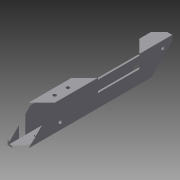
# Autodesk Inventor part: Fender Side Right
Saved by Autodesk Inventor 2015 (Build 190159000, 159)
## iProperties
Created: 2015-02-14
Part Number: Fender Side Right
Material: Generic
Document SubType Name: Modeling
Designer: chapale16
Density: 1 g/cm^3
Appearance: Default
Author: chapale16
Autodesk Inventor part; units mm, degrees
ref_plane "YZ Plane" through (0, 0, 0) normal (1, 0, 0) x (0, 1, 0)
ref_plane "XZ Plane" through (0, 0, 0) normal (0, 1, 0) x (-1, 0, 0)
ref_plane "XY Plane" through (0, 0, 0) normal (0, 0, 1) x (1, 0, 0)
sketch "Sketch1" plane through (0, 0, 0) normal (0, 0, 1) x (1, 0, 0)
  line L0 (0, 0) -> (25.4, 0)
  line L1 (25.4, 0) -> (25.4, 50.8)
  line L2 (25.4, 50.8) -> (0, 50.8)
  line L3 (0, 50.8) -> (0, 0)
  line L4 (3.175, 47.625) -> (22.225, 47.625)
  line L5 (22.225, 47.625) -> (22.225, 3.175)
  line L6 (22.225, 3.175) -> (3.175, 3.175)
  line L7 (3.175, 3.175) -> (3.175, 47.625)
  dimension "d0" = 25.4
  dimension "d1" = 50.8
  dimension "d2" = 3.175
  constraints: 16 end point, 4 parallel, 2 perpendicular, 1 horizontal, 3 other
  measures "d0" distance of L2.end L1.end
  measures "d1" distance of L1.end L0.end
  measures "d2" distance between parallel lines of L2 L4
extrude "Extrusion1" add sketch "Sketch1" along normal blind 292.1
sketch "Sketch2" plane through (0, 50.8, 0) normal (0, 1, 0) x (1, 0, 0)
  line L0 (25.4, 0) -> (25.4, -292.1) projected
  line L1 (0, 0) -> (0, -292.1) projected
  line L2 (25.4, -63.4492) -> (0, -38.0492)
  line L3 (25.4, -143.5862) -> (0, -168.9862)
  line L4 (0, -168.9862) -> (0, -38.0492)
  line L5 (25.4, -143.5862) -> (25.4, -63.4492)
  constraints: 8 end point, 4 point on line, 2 collinear
extrude "Extrusion2" cut sketch "Sketch2" against normal blind 25.4
sketch "Sketch3" plane through (25.4, 0, 0) normal (1, 0, 0) x (0, 0, -1)
  line L0 (-15.2442, 1674.64) -> (-15.2442, -147.81) projected
  line L1 (17.7758, 1674.64) -> (17.7758, -147.81) projected
  circle A0 centre (-215.7344, 12.9914) radius 3.175 projected
  circle A1 centre (-14.559, 38.1) radius 3.175 projected
  circle A2 centre (-14.559, 12.7) radius 3.175 projected
  line L2 (-34.8742, 50.8) -> (-34.8742, 25.4) projected
  line L3 (-34.8742, 25.4) -> (-169.9072, 25.4) projected
  line L4 (-169.9072, 25.4) -> (-169.9072, 50.8) projected
  line L5 (-169.9072, 50.8) -> (-234.7144, 50.8) projected
  line L6 (-234.7144, 50.8) -> (-234.7144, 0) projected
  line L7 (0, 0) -> (-234.7144, 0) projected
  line L8 (0, 50.8) -> (0, 0) projected
  line L9 (0, 50.8) -> (-34.8742, 50.8) projected
  line L10 (0, 0) -> (-292.1, 0) projected
  line L11 (-34.8742, 50.8) -> (17.7758, 50.8)
  line L12 (17.7758, 50.8) -> (17.7758, 0)
  line L13 (17.7758, 0) -> (-34.8742, 0)
  line L14 (-34.8742, 0) -> (-34.8742, 50.8)
  circle A3 centre (-18.3666, 38.1) radius 3.175
  circle A4 centre (-18.3666, 12.7) radius 3.175
  dimension "d7" = 6.35
  dimension "d8" = 6.35
  constraints: 8 end point, 2 centre point, 2 coincident, 2 parallel, 2 point on line, 1 horizontal, 1 perpendicular
  measures "d7" diameter of A3
  measures "d8" diameter of A4
extrude "Extrusion3" cut sketch "Sketch3" against normal blind 25.4 contours A3 L0 | L0 A3 A1 | A1 A3 | A4 L0 | L0 A4 A2 | A2 A4 picked at (-16.0741, 38.1) picked at (-16.0741, 12.7)
sketch "Sketch4" plane through (0, 50.8, 292.1) normal (0, 1, 0) x (1, 0, 0)
  circle A0 centre (12.7528, 77.8097) radius 3.175 projected
  circle A1 centre (-65.5643, -12.7) radius 3.175 projected
  circle A2 centre (16.4357, -12.7) radius 3.175 projected
  circle A3 centre (-65.5643, 77.8097) radius 3.175 projected
  line L0 (-75.3643, -25.3975) -> (26.2357, -25.3975) projected
  line L1 (26.2357, 88.0643) -> (26.2357, -25.3975) projected
  line L2 (26.2357, 88.0643) -> (-75.3643, 88.0643) projected
  line L3 (-75.3643, 88.0643) -> (-75.3643, -25.3975) projected
  circle A4 centre (-24.5643, 24.5643) radius 41 projected
  circle A5 centre (-24.6714, 70.0642) radius 2.55 projected
  circle A6 centre (-70.0642, 24.4572) radius 2.55 projected
  circle A7 centre (-24.4572, -20.9355) radius 2.55 projected
  circle A8 centre (20.9355, 24.6714) radius 2.55 projected
  circle A9 centre (7.5332, 56.8133) radius 2.55 projected
  circle A10 centre (7.6847, -7.5332) radius 2.55 projected
  circle A11 centre (-56.6619, -7.6847) radius 2.55 projected
  circle A12 centre (-56.8133, 56.6619) radius 2.55 projected
  circle A13 centre (-65.5643, 77.8097) radius 3.175 projected
  circle A14 centre (-65.5643, -12.7) radius 3.175 projected
  circle A15 centre (16.4357, -12.7) radius 3.175 projected
  circle A16 centre (-24.5643, 24.5643) radius 9.525 projected
  circle A17 centre (12.9268, 103.2097) radius 3.175 projected
  circle A18 centre (-78.1301, -12.7) radius 3.175 projected
  circle A19 centre (12.7528, 77.8097) radius 3.175 projected
  line L4 (25.4, -25.4) -> (-88.9, -25.4) projected
  line L5 (25.4, 123.9554) -> (25.4, -25.4) projected
  line L6 (25.4, 123.9554) -> (-88.9, 92.2721) projected
  line L7 (-88.9, -25.4) -> (-88.9, 92.2721) projected
  point P0 (0, 292.1)
extrude "Extrusion4" cut sketch "Sketch4" against normal blind 25.4 contours A0 | A17
sketch "Sketch5" plane through (25.4, 0, 0) normal (1, 0, 0) x (0, 0, -1)
  line L0 (-292.1, 0) -> (-292.1, 50.8) projected
  line L1 (0, 0) -> (-292.1, 0) projected
  point P0 (-266.7, 13.081)
  point P1 (-215.9, 13.081)
  dimension "d13" = 25.4
  dimension "d14" = 50.8
  dimension "d15" = 13.081
  dimension "d16" = 13.081
  measures "d13" distance from line of point (-266.7, 13.081) L0
  measures "d14" distance of point (-215.9, 13.081) point (-266.7, 13.081)
  measures "d15" distance from line of L1 point (-266.7, 13.081)
  measures "d16" distance from line of point (-215.9, 13.081) L1
hole "Hole1" at (25.4, 13.081, 266.7) at (25.4, 13.081, 215.9) direction (-1, 0, 0) diameter 6.35 end through all
sketch "Sketch6" plane through (0, 0, 0) normal (0, -1, 0) x (1, 0, 0)
  circle A0 centre (-24.5643, 267.5357) radius 28.3845 projected
  point P0 (0, 0)
extrude "Extrusion5" cut sketch "Sketch6" against normal blind 50.8
sketch "Sketch7" plane through (0, 50.8, 292.1) normal (0, 1, 0) x (1, 0, 0)
  line L0 (0, 10.3421) -> (0, 0) projected
  line L1 (0, 8.9261) -> (6.3676, 8.9261)
  line L2 (6.3676, 8.9261) -> (6.3676, 40.6761)
  line L3 (6.3676, 40.6761) -> (0, 40.6761)
  line L4 (0, 40.6761) -> (0, 8.9261)
  point P0 (0, 292.1)
  dimension "d26" = 31.75
  constraints: 8 end point, 2 parallel, 1 horizontal, 1 perpendicular, 1 point on line
  measures "d26" distance of L2.end L1.end
extrude "Extrusion6" cut sketch "Sketch7" against normal blind 19.05
fillet "Fillet1" radius 3.175 1 edges at (6.3676, 49.2125, 251.4239)
fillet "Fillet2" radius 3.175 1 edges at (6.3676, 49.2125, 283.1739)
sketch "Sketch8" plane through (0, 0, 0) normal (0, -1, 0) x (1, 0, 0)
  line L0 (0, 283.1739) -> (0, 292.1) projected
  line L1 (3.175, 165.8112) -> (3.175, 251.4239) projected
  line L2 (0, 284.5553) -> (3.175, 284.5553)
  line L3 (3.175, 284.5553) -> (3.175, 247.1802)
  line L4 (3.175, 247.1802) -> (0, 247.1802)
  line L5 (0, 247.1802) -> (0, 284.5553)
  point P0 (0, 0)
  constraints: 8 end point, 2 parallel, 2 point on line, 1 horizontal, 1 perpendicular
extrude "Extrusion7" add sketch "Sketch8" against normal blind 31.75
sketch "Sketch9" plane through (0, 0, 0) normal (0, -1, 0) x (1, 0, 0)
  line L0 (1.5802, 280.6086) -> (8.0596, 280.6086)
  line L1 (8.0596, 280.6086) -> (8.0596, 250.8034)
  line L2 (8.0596, 250.8034) -> (1.5802, 250.8034)
  line L3 (1.5802, 250.8034) -> (1.5802, 280.6086)
  point P0 (0, 0)
  constraints: 8 end point, 2 parallel, 1 horizontal, 1 perpendicular
extrude "Extrusion8" add sketch "Sketch9" against normal blind 3.175
body "Solid1"
